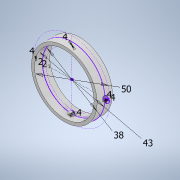
# Autodesk Inventor part: gimbal_medium_ring
Saved by Autodesk Inventor 2021 (Build 250183000, 183)
## iProperties
Created: 2021-06-14
Part Number: gimbal_medium_ring
Material: Generic
Document SubType Name: Modeling
Designer: Charlie
Density: 1 g/cm^3
Appearance: Default
Author: Charlie
Autodesk Inventor part; units mm, degrees
ref_plane "YZ Plane" through (0, 0, 0) normal (1, 0, 0) x (0, 1, 0)
ref_plane "XZ Plane" through (0, 0, 0) normal (0, 1, 0) x (-1, 0, 0)
ref_plane "XY Plane" through (0, 0, 0) normal (0, 0, 1) x (1, 0, 0)
sketch "Sketch1" plane through (0, 0, 0) normal (0, 0, 1) x (1, 0, 0)
  circle A0 centre (0, 0) radius 25 construction
  circle A1 centre (0, 0) radius 21.5
  circle A2 centre (0, 0) radius 19.5
  circle A3 centre (0, 0) radius 19 construction
  circle A4 centre (0, 0) radius 17 construction
  line L0 (25, 0) -> (-25, 0) construction
  line L1 (0, 25) -> (0, -25) construction
  circle A5 centre (-23, 0) radius 2 construction
  circle A6 centre (23, 0) radius 2 construction
  circle A7 centre (0, 19.5) radius 2
  circle A8 centre (0, -19.5) radius 2
  line L2 (-25, 0) -> (-21, 0)
  line L3 (21, 0) -> (25, 0)
  line L4 (0, 21.5) -> (0, 17.5)
  line L5 (0, -17.5) -> (0, -21.5)
  circle A9 centre (22.4059, 0) radius 2
  circle A10 centre (-22.4059, 0) radius 2
  line L6 (-24.4059, 0) -> (-20.4059, 0)
  line L7 (24.4059, 0) -> (20.4059, 0)
  dimension "d6" = 4
  dimension "d0" = 50
  dimension "d2" = 43
  dimension "d3" = 2
  dimension "d4" = 38
  dimension "d5" = 2
  dimension "d7" = 4
  dimension "d8" = 4
  dimension "d9" = 4
  dimension "d22" = 4
  constraints: 17 point on circle, 16 end point, 14 point on line, 10 centre point, 3 coincident, 1 horizontal, 1 midpoint, 1 perpendicular, 1 symmetric about line, 5 other
  measures "d0" diameter of A0
  measures "d2" diameter of A1
  measures "d3" radial gap between concentric circles of A1 A2
  measures "d4" diameter of A3
  measures "d5" radial gap between concentric circles of A3 A4
  measures "d7" diameter of A6
  measures "d8" diameter of A7
  measures "d9" diameter of A8
  measures "d22" diameter of A9
extrude "Extrusion1" add sketch "Sketch1" along normal mid plane 10 contours L3 L7 A9 A1 | A1 A9 L7 L3 | A9 A1 A8 A2 A7 | A7 A2 A8 A1 A10 | L4 A2 A7 | A7 A2 L4 | L5 A2 A8 | A8 A2 L5 | A10 L6 L2 A1 | A1 L2 L6 A10 picked at (-0.5203, 20.0925) picked at (0.5115, 20.0968) picked at (0.5115, -20.0968) picked at (-0.5203, -20.0925)
revolve "Revolution1" cut sketch "Sketch1" angle 360 about axis through (-25, 0, 0) along (1, 0, 0) picked at (-22.396, -0.4915) picked at (-21.0251, -0.4685) contours A10 L2 A1 | A1 L2 L6 A10
revolve "Revolution2" cut sketch "Sketch1" angle 360 about axis through (21, 0, 0) along (1, 0, 0) picked at (22.396, -0.4915) picked at (21.0251, -0.4685) contours L3 A9 A1 | A1 A9 L7 L3
revolve "Revolution3" add sketch "Sketch1" angle 360 about axis through (0, 25, 0) along (0, -1, 0) picked at (-0.5203, 20.0925) picked at (-0.3659, 18.8452) contours L4 A2 A7 | A2 L4 A7
revolve "Revolution4" add sketch "Sketch1" angle 360 about axis through (0, 25, 0) along (0, -1, 0) picked at (-0.5203, -20.0925) picked at (-0.3659, -18.8452) contours A8 A2 L5 | A8 L5 A2
body "Solid1"
